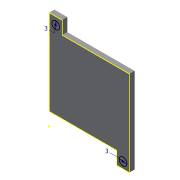
# Autodesk Inventor part: 00_cellstorm_Amplifier
Saved by Autodesk Inventor 2019 (Build 230136000, 136)
## iProperties
Created: 2020-05-04
Part Number: 00_cellstorm_Amplifier
Material: Generic
Document SubType Name: Modeling
Designer: diederichbenedict
Density: 1 g/cm^3
Appearance: Default
Author: diederichbenedict
Autodesk Inventor part; units mm, degrees
ref_plane "YZ Plane" through (0, 0, 0) normal (1, 0, 0) x (0, 1, 0)
ref_plane "XZ Plane" through (0, 0, 0) normal (0, 1, 0) x (-1, 0, 0)
ref_plane "XY Plane" through (0, 0, 0) normal (0, 0, 1) x (1, 0, 0)
sketch "Sketch1" plane through (0, 0, 0) normal (0, 0, 1) x (1, 0, 0)
  line L0 (0, 0) -> (31, 0)
  line L1 (31, 0) -> (31, 38)
  line L2 (31, 38) -> (0, 38)
  line L3 (0, 38) -> (0, 0)
  line L4 (31, 38) -> (5, 38)
  line L5 (5, 38) -> (5, 33)
  line L6 (5, 33) -> (31, 33)
  line L7 (31, 33) -> (31, 38)
  line L8 (0, 0) -> (26, 0)
  line L9 (26, 0) -> (26, 5)
  line L10 (26, 5) -> (0, 5)
  line L11 (0, 5) -> (0, 0)
  dimension "d0" = 31
  dimension "d1" = 38
  dimension "d3" = 5
  dimension "d4" = 5
  dimension "d5" = 5
  dimension "d6" = 5
  constraints: 24 end point, 6 parallel, 3 horizontal, 3 perpendicular
  measures "d0" distance of L2.end L1.end
  measures "d1" distance of L1.end L0.end
  measures "d3" distance of L5.end L4.end
  measures "d4" distance of L9.end L8.end
  measures "d5" distance between parallel lines of L9 L1
  measures "d6" distance between parallel lines of L3 L5
extrude "Extrusion1" add sketch "Sketch1" along normal blind 2 contours L9 L10 L3 L2 L5 L6 L1 L0
sketch "Sketch2" plane through (0, 0, 2) normal (0, 0, 1) x (1, 0, 0)
  line L0 (26, 5) -> (26, 0) projected
  line L1 (26, 0) -> (31, 0) projected
  line L2 (31, 0) -> (31, 33) projected
  line L3 (31, 33) -> (5, 33) projected
  line L4 (5, 33) -> (5, 38) projected
  line L5 (5, 38) -> (0, 38) projected
  line L6 (0, 38) -> (0, 5) projected
  line L7 (0, 5) -> (26, 5) projected
  circle A0 centre (2.5, 35.0921) radius 1.5
  circle A1 centre (28.5, 2.5) radius 1.5
  point P0 (0, 0)
  dimension "d9" = 3
  dimension "d10" = 3
  constraints: 2 centre point
  measures "d9" diameter of A0
  measures "d10" diameter of A1
extrude "Extrusion2" cut sketch "Sketch2" against normal blind 2 contours A0 | A1
body "Solid1"
